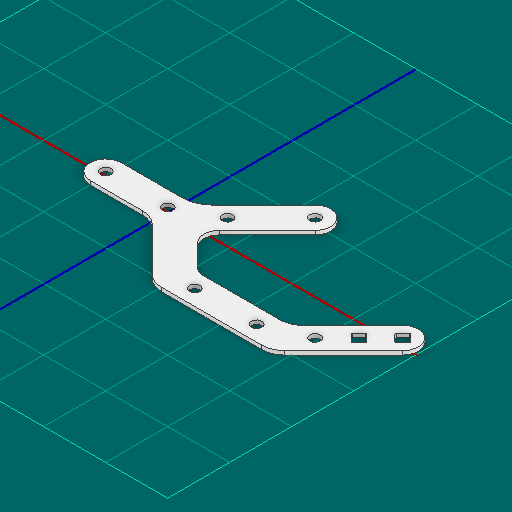
# Autodesk Inventor part: join_gusset
Saved by Autodesk Inventor 2025 (Build 290162000, 162)
## iProperties
Created: 2024-08-17
Part Number: join_gusset
Material: Acetal Resin, White
Document SubType Name: Modeling
Designer: averey
Density: 1.425 g/cm^3
Appearance: Smooth - White
d5: 0.500 in
d6: 135.00 deg
d7: 0.375 in
d8: 0.500 in
d9: 0.375 in
d10: 0.375 in
d11: 0.500 in
d12: 0.188 in
d15: 1.250 in
d16: 0.500 in
d17: 45.00 deg
d18: 0.250 in
d19: 0.172 in
d20: 0.250 in
d24: 0.172 in
Author: averey
Autodesk Inventor part; units mm, degrees
ref_plane "YZ Plane" through (0, 0, 0) normal (1, 0, 0) x (0, 1, 0)
ref_plane "XZ Plane" through (0, 0, 0) normal (0, 1, 0) x (-1, 0, 0)
ref_plane "XY Plane" through (0, 0, 0) normal (0, 0, 1) x (1, 0, 0)
sketch "main" plane through (0, 0, 0) normal (0, 0, 1) x (1, 0, 0)
  line L0 (-25.7346, 15.6158) -> (-23.1842, 13.0654)
  arc A0 (-23.1842, 12.347) -> (-23.1842, 13.0654) centre (-23.5434, 12.7062) ccw
  line L1 (-23.1842, 12.347) -> (-25.7346, 9.7966)
  line L2 (-29.0034, 13.0654) -> (-26.453, 15.6158)
  circle A1 centre (-26.0938, 12.7062) radius 2.1844 construction
  arc A2 (-29.0034, 13.0654) -> (-29.0034, 12.347) centre (-28.6442, 12.7062) ccw
  line L3 (-26.453, 9.7966) -> (-29.0034, 12.347)
  arc A3 (-32.1645, 3.3667) -> (-32.1645, 4.0851) centre (-32.5237, 3.7259) ccw
  arc A4 (-26.453, 9.7966) -> (-25.7346, 9.7966) centre (-26.0938, 10.1558) ccw
  arc A5 (-8.6781, 35.1568) -> (-15.4133, 32.367) centre (-8.6781, 25.6318) ccw
  circle A6 centre (-17.1136, 21.6864) radius 2.1844
  arc A7 (-25.7346, 15.6158) -> (-26.453, 15.6158) centre (-26.0938, 15.2566) ccw
  line L4 (-10.1527, 19.667) -> (-30.584, -0.7642)
  line L5 (-39.5642, 8.216) -> (-15.4133, 32.367)
  line L6 (-17.1136, 21.6864) -> (-10.7636, 21.6864) construction
  line L7 (-17.1136, 21.6864) -> (-21.6037, 26.1765)
  arc A8 (-34.7149, 6.6355) -> (-35.4333, 6.6355) centre (-35.0741, 6.2763) ccw
  line L8 (-34.7149, 6.6355) -> (-32.1645, 4.0851)
  line L9 (-32.1645, 3.3667) -> (-34.7149, 0.8163)
  arc A9 (-37.9837, 4.0851) -> (-37.9837, 3.3667) centre (-37.6245, 3.7259) ccw
  arc A10 (-35.4333, 0.8163) -> (-34.7149, 0.8163) centre (-35.0741, 1.1755) ccw
  line L10 (-35.4333, 0.8163) -> (-37.9837, 3.3667)
  arc A11 (-39.5642, 8.216) -> (-30.584, -0.7642) centre (-35.0741, 3.7259) ccw
  line L11 (-37.9837, 4.0851) -> (-35.4333, 6.6355)
  circle A12 centre (43.5032, -3.0093) radius 2.1844
  circle A13 centre (25.5426, -20.9698) radius 2.1844
  arc A14 (21.0525, -16.4797) -> (30.0328, -25.4599) centre (25.5426, -20.9698) ccw
  line L12 (21.0525, -16.4797) -> (40.6569, 3.1247)
  line L13 (50.966, -4.5267) -> (30.0328, -25.4599)
  circle A15 centre (59.4482, 5.5431) radius 2.1844
  line L14 (72.1482, 11.8931) -> (63.3936, 11.8931)
  line L15 (56.6584, 14.6829) -> (38.9743, 32.367)
  line L16 (72.1482, -0.8069) -> (59.9463, -0.8069)
  arc A16 (56.6584, 14.6829) -> (63.3936, 11.8931) centre (63.3936, 21.4181) ccw
  line L17 (84.8482, 11.8931) -> (72.1482, 11.8931)
  line L18 (84.8482, -0.8069) -> (72.1482, -0.8069)
  circle A17 centre (84.8482, 5.5431) radius 2.1844
  arc A18 (84.8482, -0.8069) -> (84.8482, 11.8931) centre (84.8482, 5.5431) ccw
  arc A19 (59.9463, -0.8069) -> (50.966, -4.5267) centre (59.9463, -13.5069) ccw
  arc A20 (-3.4175, 22.4568) -> (-10.1527, 19.667) centre (-3.4175, 12.9318) ccw
  line L19 (-3.4175, 22.4568) -> (28.3325, 22.4568)
  line L20 (-8.6781, 35.1568) -> (32.2391, 35.1568)
  arc A21 (31.7001, 21.0619) -> (28.3325, 22.4568) centre (28.3325, 17.6943) ccw
  arc A22 (38.9743, 32.367) -> (32.2391, 35.1568) centre (32.2391, 25.6318) ccw
  line L21 (31.7001, 21.0619) -> (40.6569, 12.105)
  line L22 (31.7001, 21.0619) -> (44.367, 21.0619) construction
  arc A23 (40.6569, 3.1247) -> (40.6569, 12.105) centre (36.1668, 7.6149) ccw
  circle A24 centre (25.1575, 28.8068) radius 2.1844
  circle A25 centre (-0.2425, 28.8068) radius 2.1844
  point P0 (7.2046, 10.3806)
  point P1 (59.4482, 11.8931)
  dimension "d5" = 12.7
  dimension "d6" = 135
  dimension "d7" = 9.525
  dimension "d8" = 12.7
  dimension "d9" = 9.525
  dimension "d10" = 9.525
  dimension "d11" = 12.7
  dimension "d12" = 4.7625
  dimension "d15" = 31.75
  dimension "d16" = 12.7
  dimension "d17" = 45
  dimension "d18" = 6.35
  dimension "d19" = 4.3688
  dimension "d20" = 6.35
  dimension "d24" = 4.3688
  measures "d5" diameter of A14
  measures "d6" angle of L6 L7
  measures "d7" radius of A22
  measures "d8" distance between parallel lines of L13 L12
  measures "d9" radius of A20
  measures "d10" radius of A16
  measures "d11" radius of A19
  measures "d12" radius of A21
  measures "d15" distance of L19.start L19.end
  measures "d16" distance between parallel lines of L20 L19
  measures "d17" angle of L21 L22
  measures "d18" radius of A23
  measures "d19" diameter of A24
  measures "d20" distance from line of L19 A24.centre
  measures "d24" diameter of A25
sketch "Sketch1" plane through (0, 0, 0) normal (0, 1, 0) x (-1, 0, 0)
  line L0 (-85.1829, 10.0727) -> (-82.6325, 7.5223)
  arc A0 (-82.6325, 6.8039) -> (-82.6325, 7.5223) centre (-82.9917, 7.1631) ccw
  line L1 (-82.6325, 6.8039) -> (-85.1829, 4.2535)
  line L2 (-88.4517, 7.5223) -> (-85.9013, 10.0727)
  circle A1 centre (-85.5421, 7.1631) radius 2.1844 construction
  arc A2 (-88.4517, 7.5223) -> (-88.4517, 6.8039) centre (-88.0925, 7.1631) ccw
  line L3 (-85.9013, 4.2535) -> (-88.4517, 6.8039)
  arc A3 (-91.6127, -2.1764) -> (-91.6127, -1.4579) centre (-91.9719, -1.8171) ccw
  arc A4 (-85.9013, 4.2535) -> (-85.1829, 4.2535) centre (-85.5421, 4.6127) ccw
  arc A5 (-68.1263, 29.6137) -> (-74.8615, 26.8239) centre (-68.1263, 20.0887) ccw
  circle A6 centre (-76.5618, 16.1434) radius 2.1844
  arc A7 (-85.1829, 10.0727) -> (-85.9013, 10.0727) centre (-85.5421, 9.7135) ccw
  line L4 (-69.601, 14.1239) -> (-90.0322, -6.3073)
  line L5 (-99.0125, 2.673) -> (-74.8615, 26.8239)
  line L6 (-76.5618, 16.1434) -> (-70.2118, 16.1434) construction
  line L7 (-76.5618, 16.1434) -> (-81.0519, 20.6335)
  arc A8 (-94.1631, 1.0925) -> (-94.8815, 1.0925) centre (-94.5223, 0.7332) ccw
  line L8 (-94.1631, 1.0925) -> (-91.6127, -1.4579)
  line L9 (-91.6127, -2.1764) -> (-94.1631, -4.7268)
  arc A9 (-97.4319, -1.4579) -> (-97.4319, -2.1764) centre (-97.0727, -1.8171) ccw
  arc A10 (-94.8815, -4.7268) -> (-94.1631, -4.7268) centre (-94.5223, -4.3675) ccw
  line L10 (-94.8815, -4.7268) -> (-97.4319, -2.1764)
  arc A11 (-99.0125, 2.673) -> (-90.0322, -6.3073) centre (-94.5223, -1.8172) ccw
  line L11 (-97.4319, -1.4579) -> (-94.8815, 1.0925)
  circle A12 centre (-15.9451, -8.5524) radius 2.1844
  circle A13 centre (-33.9056, -26.5129) radius 2.1844
  arc A14 (-38.3957, -22.0227) -> (-29.4155, -31.003) centre (-33.9056, -26.5129) ccw
  line L12 (-38.3957, -22.0227) -> (-18.7913, -2.4183)
  line L13 (-8.4822, -10.0697) -> (-29.4155, -31.003)
  circle A15 centre (0, 0) radius 2.1844
  line L14 (12.7, 6.35) -> (3.9454, 6.35)
  line L15 (-2.7898, 9.1398) -> (-20.4739, 26.8239)
  line L16 (12.7, -6.35) -> (0.498, -6.35)
  arc A16 (-2.7898, 9.1398) -> (3.9454, 6.35) centre (3.9454, 15.875) ccw
  line L17 (25.4, 6.35) -> (12.7, 6.35)
  line L18 (25.4, -6.35) -> (12.7, -6.35)
  circle A17 centre (25.4, 0) radius 2.1844
  arc A18 (25.4, -6.35) -> (25.4, 6.35) centre (25.4, 0) ccw
  arc A19 (0.498, -6.35) -> (-8.4822, -10.0697) centre (0.498, -19.05) ccw
  arc A20 (-62.8658, 16.9137) -> (-69.601, 14.1239) centre (-62.8658, 7.3887) ccw
  line L19 (-62.8658, 16.9137) -> (-31.1158, 16.9137)
  line L20 (-68.1263, 29.6137) -> (-27.2091, 29.6137)
  arc A21 (-27.7482, 15.5188) -> (-31.1158, 16.9137) centre (-31.1158, 12.1512) ccw
  arc A22 (-20.4739, 26.8239) -> (-27.2091, 29.6137) centre (-27.2091, 20.0887) ccw
  line L21 (-27.7482, 15.5188) -> (-18.7913, 6.5619)
  line L22 (-27.7482, 15.5188) -> (-15.0812, 15.5188) construction
  arc A23 (-18.7913, -2.4183) -> (-18.7913, 6.5619) centre (-23.2814, 2.0718) ccw
  circle A24 centre (-34.2908, 23.2637) radius 2.1844
  circle A25 centre (-59.6908, 23.2637) radius 2.1844
  constraints: 2 other
extrude "Extrusion1" add sketch "Sketch1" along normal blind 1.5875
body "Solid1"
